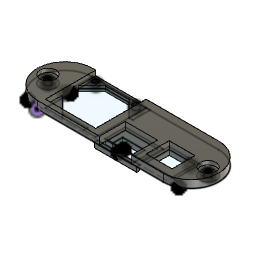
Complete_Housing_MyStat (Autodesk Fusion 360 archive; units mm, degrees)
design "MyStat Back Panel"
Autodesk Fusion 360 part; units mm, degrees
sketch "Sketch1" plane through (0, 0, 0) normal (0, 0, 1) x (1, 0, 0)
  line L0 (0, 0) -> (50, 0)
  line L1 (0, 22) -> (50, 22)
  arc A0 (0, 22) -> (0, 0) centre (0, 11) ccw
  arc A1 (50, 0) -> (50, 22) centre (50, 11) ccw
  circle A2 centre (-6.775, 11) radius 1.225
  circle A3 centre (56.775, 11) radius 1.225
  line L2 (-5, 1.202) -> (55, 1.202) construction
  line L3 (40.05, 12.3) -> (50.3, 12.3)
  line L4 (50.3, 12.3) -> (50.3, 3.2)
  line L5 (50.3, 3.2) -> (40.05, 3.2)
  line L6 (40.05, 3.2) -> (40.05, 12.3)
  line L7 (26.7, 7.2) -> (35.5, 7.2)
  line L8 (35.5, 7.2) -> (35.5, 3.2)
  line L9 (35.5, 3.2) -> (26.7, 3.2)
  line L10 (26.7, 3.2) -> (26.7, 7.2)
  line L11 (24.7, 3.2) -> (37.5, 3.2)
  line L12 (37.5, 3.2) -> (37.5, 10.2)
  line L13 (37.5, 10.2) -> (24.7, 10.2)
  line L14 (24.7, 10.2) -> (24.7, 3.2)
  line L15 (39.05, 3.2) -> (51.3, 3.2)
  line L16 (51.3, 3.2) -> (51.3, 13.3)
  line L17 (51.3, 13.3) -> (39.05, 13.3)
  line L18 (39.05, 13.3) -> (39.05, 3.2)
  line L19 (24.7, 1.202) -> (37.5, 1.202)
  line L20 (37.5, 1.202) -> (37.5, 0)
  line L21 (37.5, 0) -> (24.7, 0)
  line L22 (24.7, 0) -> (24.7, 1.202)
  line L23 (22.7, 1.202) -> (22.7, 0)
  line L24 (39.5, 1.202) -> (39.5, 0)
  line L25 (22.7, 1.202) -> (24.7, 1.202)
  line L26 (37.5, 1.202) -> (39.5, 1.202)
  line L27 (23.7, 3.2) -> (38.5, 3.2)
  line L28 (38.5, 3.2) -> (38.5, 11.2)
  line L29 (38.5, 11.2) -> (23.7, 11.2)
  line L30 (23.7, 11.2) -> (23.7, 3.2)
  line L31 (24.7, 3.2) -> (24.7, 1.202)
  line L32 (37.5, 3.2) -> (37.5, 1.202)
  line L33 (38.5, 3.2) -> (39.05, 3.2)
  line L34 (38.5, 11.2) -> (39.05, 11.2)
  circle A4 centre (-6.775, 11) radius 3.125
  circle A5 centre (56.775, 11) radius 3.125
  line L35 (1.2, 22) -> (21.2, 22)
  line L36 (21.2, 22) -> (21.2, 2)
  line L37 (21.2, 2) -> (1.2, 2)
  line L38 (1.2, 2) -> (1.2, 22)
  line L39 (7.9882, 22) -> (1.2, 15.2118)
  line L40 (14.4118, 22) -> (21.2, 15.2118)
  circle A6 centre (3.2, 20) radius 1.25
  circle A7 centre (19.2, 20) radius 1.25
  line L41 (6.4882, 20.5) -> (15.9118, 20.5)
  line L42 (21.2, 15.2118) -> (22.7, 15.2118)
  line L43 (22.7, 15.2118) -> (22.7, 22)
  line L44 (22.7, 22) -> (21.2, 22)
  line L45 (21.2, 22) -> (21.2, 15.2118)
  line L46 (1.2, 15.2118) -> (-0.3, 15.2118)
  line L47 (-0.3, 15.2118) -> (-0.3, 21.9959)
  line L48 (-0.3, 21.9959) -> (1.2, 21.9959)
  line L49 (1.2, 21.9959) -> (1.2, 15.2118)
  line L50 (1.2, 8.7882) -> (7.9882, 2)
  line L51 (6.4882, 3.5) -> (16.4882, 3.5)
  line L52 (16.4882, 3.5) -> (16.4882, 2)
  point P0 (-5, 1.202)
  point P1 (55, 1.202)
  point P2 (31.1, 1.202)
  point P3 (31.1, 3.2)
  point P4 (1.2, 12)
  dimension "d1" = 50
  dimension "d2" = 22
  dimension "d3" = 2.45
  dimension "d5" = 2.45
  dimension "d11" = 60
  dimension "d12" = 9.1
  dimension "d13" = 10.25
  dimension "d16" = 4.7
  dimension "d17" = 8.8
  dimension "d18" = 4
  dimension "d20" = 19.5
  dimension "d51" = 3
  dimension "d52" = 2
  dimension "d53" = 2
  dimension "d54" = 1
  dimension "d55" = 1
  dimension "d56" = 1
  dimension "d57" = 12.8
  dimension "d58" = 2
  dimension "d59" = 2
  dimension "d60" = 1
  dimension "d61" = 1
  dimension "d62" = 1
  dimension "d75" = 6.775
  dimension "d76" = 6.775
  dimension "d77" = 6.25
  dimension "d78" = 6.25
  dimension "d81" = 3.2
  dimension "d82" = 3.2
  dimension "d89" = 20
  dimension "d90" = 20
  dimension "d91" = 2.5
  dimension "d98" = 4.8
  dimension "d99" = 4.8
  dimension "d100" = 45
  dimension "d101" = 45
  dimension "d102" = 2.5
  dimension "d103" = 2.5
  dimension "d104" = 2
  dimension "d105" = 2
  dimension "d106" = 2
  dimension "d107" = 2
  dimension "d110" = 1.5
  dimension "d111" = 1.5
  dimension "d112" = 1.5
  dimension "d118" = 45
  dimension "d119" = 4.8
  dimension "d120" = 10
  dimension "d121" = 1.5
  constraint coincident L0.start A0.end
  constraint horizontal L0
  constraint horizontal L1
  constraint tangent L0 A0
  constraint tangent L1 A0
  constraint tangent L0 A1
  constraint tangent L1 A1
  constraint horizontal A0.centre A2.centre
  constraint horizontal A1.centre A3.centre
  constraint coincident A0 P0
  constraint coincident A1 P1
  constraint coincident P0 L2.start
  constraint coincident P1 L2.end
  constraint horizontal L2
  constraint horizontal L3
  constraint vertical L4
  constraint horizontal L5
  constraint vertical L6
  constraint horizontal L7
  constraint vertical L8
  constraint horizontal L9
  constraint vertical L10
  constraint horizontal L11
  constraint vertical L12
  constraint horizontal L13
  constraint vertical L14
  constraint collinear L9 L11
  constraint horizontal L15
  constraint vertical L16
  constraint horizontal L17
  constraint vertical L18
  constraint collinear L5 L15
  constraint horizontal L19
  constraint vertical L20
  constraint horizontal L21
  constraint vertical L22
  constraint coincident L0 L20.end
  constraint coincident L2 L19.start
  constraint midpoint L19 P2
  constraint midpoint L9 P3
  constraint vertical P2 P3
  constraint coincident L2 L23.start
  constraint coincident L0 L23.end
  constraint perpendicular L0 L23
  constraint coincident L2 L24.start
  constraint coincident L0 L24.end
  constraint perpendicular L0 L24
  constraint horizontal L27
  constraint vertical L28
  constraint horizontal L29
  constraint vertical L30
  constraint collinear L9 L27
  constraint coincident L18 L34.end
  constraint perpendicular L18 L34
  constraint concentric A2 A4
  constraint concentric A3 A5
  constraint horizontal L35
  constraint vertical L36
  constraint horizontal L37
  constraint vertical L38
  constraint coincident L35 L39.start
  constraint coincident L38 L39.end
  constraint coincident L35 L40.start
  constraint coincident L36 L40.end
  constraint collinear L1 L35
  constraint midpoint L38 P4
  constraint coincident L39 L41.start
  constraint coincident L40 L41.end
  constraint perpendicular L36 L41
  constraint horizontal L42
  constraint vertical L43
  constraint horizontal L44
  constraint vertical L45
  constraint coincident L1 L43.end
  constraint horizontal L46
  constraint vertical L47
  constraint horizontal L48
  constraint vertical L49
  constraint coincident A0 L47.end
  constraint coincident L38 L50.start
  constraint coincident L37 L50.end
  constraint coincident L50 L51.start
  constraint perpendicular L36 L51
  constraint coincident L37 L52.end
  constraint perpendicular L37 L52
  measures "d1" distance of L0.start L0.end
  measures "d2" distance of L0 L1
  measures "d3" diameter of A2
  measures "d5" diameter of A3
  measures "d11" distance of P0 P1
  measures "d12" distance of L3 L5
  measures "d13" distance of L4 L6
  measures "d16" distance of P1 L4
  measures "d17" distance of L7.start L7.end
  measures "d18" distance of L7.start L9.end
  measures "d20" distance of P1 L8
  measures "d51" distance of L7 L13
  measures "d52" distance of L10 L14
  measures "d53" distance of L8 L12
  measures "d54" distance of L6 L18
  measures "d55" distance of L3 L17
  measures "d56" distance of L4 L16
  measures "d57" distance of L20 L22
  measures "d58" distance of L22 L23
  measures "d59" distance of L20 L24
  measures "d60" distance of L14 L30
  measures "d61" distance of L13 L29
  measures "d62" distance of L12 L28
  measures "d75" distance of A0.centre A2.centre
  measures "d76" distance of A1.centre A3.centre
  measures "d77" diameter of A4
  measures "d78" diameter of A5
  measures "d81" distance of L0 L9
  measures "d82" distance of L0 L5
  measures "d89" distance of L35.start L35.end
  measures "d90" distance of L35.start L37.end
  measures "d91" distance of L30 L36
  measures "d98" distance of L35.start L39
  measures "d99" distance of L35.end L40
  measures "d100" angle of L38 L39
  measures "d101" angle of L36 L40
  measures "d102" diameter of A6
  measures "d103" diameter of A7
  measures "d104" distance of L38 A6.centre
  measures "d105" distance of L35 A6.centre
  measures "d106" distance of L35 A7.centre
  measures "d107" distance of L36 A7.centre
  measures "d110" distance of L1 L41
  measures "d111" distance of L40.end L42.end
  measures "d112" distance of L39.end L46.end
  measures "d118" angle of L37 L50
  measures "d119" distance of L37.end L50
  measures "d120" distance of L51.start L51.end
  measures "d121" distance of L51.end L52.end
extrude "Extrude16" add sketch "Sketch1" along normal blind 3 contours L0 L1 A0 A1 L5 L15 L16 L17 L18 L23 L24 L25 L26 L27 L29 L30 L31 L32 L33 L34 L36 L37 L38 L42 L43 L46 L47 | L0 L22 L23 L25 | L38 L46 L47 L48 L49 | L1 A0 L38 L48 | L1 L35 L38 L39 L49 | L0 L20 L24 L26 | L36 L37 L38 L39 L40 L41 L50 L51 L52 | L12 L13 L14 L27 L28 L29 L30 | L1 L35 L39 L40 L41 | L37 L38 L50 | L1 L35 L36 L40 L45 | L37 L50 L51 L52 | L18 L28 L33 L34 | L1 L36 L42 L43 L44 L45 | L3 L4 L6 L15 L16 L17 L18 | A6 | A7
extrude "Extrude17" add sketch "Sketch1" against normal blind 2 contours L0 L22 L23 L25 | L0 L19 L20 L21 L22 | L0 L20 L24 L26 | L7 L8 L10 L11 L12 L13 L14 L27 | L12 L13 L14 L27 L28 L29 L30 | L3 L4 L6 L15 L16 L17 L18
extrude "Extrude18" add sketch "Sketch1" along normal blind 1.5 contours A4 | A5
extrude "Extrude19" cut sketch "Sketch1" along normal blind 3 contours L1 L35 L38 L39 L49 | L36 L37 L38 L39 L40 L41 L50 L51 L52 | L1 L35 L39 L40 L41 | L37 L38 L50 | L1 L35 L36 L40 L45 | L37 L50 L51 L52 | A6 | A7
extrude "Extrude20" add sketch "Sketch1" along normal blind 1 and the other way blind 1 contours L1 L35 L38 L39 L49 | L1 L35 L39 L40 L41 | L1 L35 L36 L40 L45
extrude "Extrude21" add sketch "Sketch1" against normal blind 1 contours L38 L46 L47 L48 L49 | L1 L36 L42 L43 L44 L45
extrude "Extrude23" add sketch "Sketch1" along normal blind 1 contours L37 L38 L50 | L37 L50 L51 L52
equation "d76 = d75"
equation "d82 = d81"

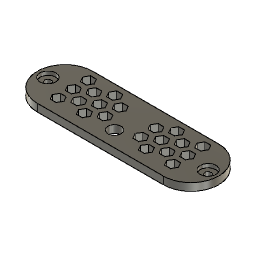
design "MyStat Front Panel 2.5"
Autodesk Fusion 360 part; units mm, degrees
sketch "Sketch1" plane through (0, 0, 0) normal (0, 0, 1) x (1, 0, 0)
  line L0 (0, 0) -> (50, 0)
  line L1 (0, 22) -> (50, 22)
  arc A0 (0, 22) -> (0, 0) centre (0, 11) ccw
  arc A1 (50, 0) -> (50, 22) centre (50, 11) ccw
  circle A2 centre (-6.775, 11) radius 1.225
  circle A3 centre (56.775, 11) radius 1.225
  circle A4 centre (24.5, 6.15) radius 2.6
  line L2 (-5, 1.202) -> (55, 1.202) construction
  circle A5 centre (-6.775, 11) radius 3.125
  circle A6 centre (56.775, 11) radius 3.125
  line L3 (4.6188, 18) -> (3.4641, 20)
  line L4 (3.4641, 20) -> (1.1547, 20)
  line L5 (1.1547, 20) -> (0, 18)
  line L6 (0, 18) -> (1.1547, 16)
  line L7 (1.1547, 16) -> (3.4641, 16)
  line L8 (3.4641, 16) -> (4.6188, 18)
  line L9 (0, 22) -> (0, 0) construction
  line L10 (50, 22) -> (50, 0) construction
  line L11 (4.6188, 12) -> (3.4641, 14)
  line L12 (3.4641, 14) -> (1.1547, 14)
  line L13 (1.1547, 10) -> (3.4641, 10)
  line L14 (3.4641, 10) -> (4.6188, 12)
  line L15 (1.1547, 14) -> (0, 12)
  line L16 (0, 12) -> (1.1547, 10)
  line L17 (4.6188, 6) -> (3.4641, 8)
  line L18 (3.4641, 8) -> (1.1547, 8)
  line L19 (1.1547, 4) -> (3.4641, 4)
  line L20 (3.4641, 4) -> (4.6188, 6)
  line L21 (1.1547, 8) -> (0, 6)
  line L22 (0, 6) -> (1.1547, 4)
  line L23 (9.815, 15) -> (8.6603, 17)
  line L24 (8.6603, 17) -> (6.3509, 17)
  line L25 (6.3509, 13) -> (8.6603, 13)
  line L26 (8.6603, 13) -> (9.815, 15)
  line L27 (6.3509, 17) -> (5.1962, 15)
  line L28 (5.1962, 15) -> (6.3509, 13)
  line L29 (9.815, 9) -> (8.6603, 11)
  line L30 (8.6603, 11) -> (6.3509, 11)
  line L31 (6.3509, 7) -> (8.6603, 7)
  line L32 (8.6603, 7) -> (9.815, 9)
  line L33 (6.3509, 11) -> (5.1962, 9)
  line L34 (5.1962, 9) -> (6.3509, 7)
  line L35 (15.0111, 12) -> (13.8564, 14)
  line L36 (13.8564, 14) -> (11.547, 14)
  line L37 (11.547, 10) -> (13.8564, 10)
  line L38 (13.8564, 10) -> (15.0111, 12)
  line L39 (11.547, 14) -> (10.3923, 12)
  line L40 (10.3923, 12) -> (11.547, 10)
  line L41 (15.0111, 6) -> (13.8564, 8)
  line L42 (11.547, 4) -> (13.8564, 4)
  line L43 (11.547, 8) -> (10.3923, 6)
  line L44 (13.8564, 8) -> (11.547, 8)
  line L45 (10.3923, 6) -> (11.547, 4)
  line L46 (13.8564, 4) -> (15.0111, 6)
  line L47 (20.2073, 15) -> (19.0526, 17)
  line L48 (16.7432, 13) -> (19.0526, 13)
  line L49 (16.7432, 17) -> (15.5885, 15)
  line L50 (19.0526, 17) -> (16.7432, 17)
  line L51 (15.5885, 15) -> (16.7432, 13)
  line L52 (19.0526, 13) -> (20.2073, 15)
  line L53 (15.0111, 18) -> (13.8564, 20)
  line L54 (11.547, 16) -> (13.8564, 16)
  line L55 (11.547, 20) -> (10.3923, 18)
  line L56 (13.8564, 20) -> (11.547, 20)
  line L57 (10.3923, 18) -> (11.547, 16)
  line L58 (13.8564, 16) -> (15.0111, 18)
  line L59 (15.5885, 9) -> (16.7432, 7)
  line L60 (19.0526, 7) -> (20.2073, 9)
  line L61 (16.7432, 11) -> (15.5885, 9)
  line L62 (19.0526, 11) -> (16.7432, 11)
  line L63 (20.2073, 9) -> (19.0526, 11)
  line L64 (16.7432, 7) -> (19.0526, 7)
  line L65 (25, 22) -> (25, 0) construction
  line L66 (50, 6) -> (48.8453, 4)
  line L67 (48.8453, 4) -> (46.5359, 4)
  line L68 (46.5359, 14) -> (48.8453, 14)
  line L69 (41.3397, 11) -> (43.6491, 11)
  line L70 (38.453, 10) -> (36.1436, 10)
  line L71 (48.8453, 16) -> (46.5359, 16)
  line L72 (48.8453, 10) -> (46.5359, 10)
  line L73 (40.185, 9) -> (41.3397, 11)
  line L74 (36.1436, 8) -> (38.453, 8)
  line L75 (33.2568, 7) -> (30.9474, 7)
  line L76 (48.8453, 20) -> (50, 18)
  line L77 (50, 12) -> (48.8453, 10)
  line L78 (33.2568, 13) -> (30.9474, 13)
  line L79 (30.9474, 13) -> (29.7927, 15)
  line L80 (30.9474, 7) -> (29.7927, 9)
  line L81 (30.9474, 11) -> (33.2568, 11)
  line L82 (41.3397, 7) -> (40.185, 9)
  line L83 (46.5359, 8) -> (48.8453, 8)
  line L84 (29.7927, 15) -> (30.9474, 17)
  line L85 (29.7927, 9) -> (30.9474, 11)
  line L86 (34.9889, 6) -> (36.1436, 8)
  line L87 (46.5359, 20) -> (48.8453, 20)
  line L88 (43.6491, 7) -> (41.3397, 7)
  line L89 (33.2568, 11) -> (34.4115, 9)
  line L90 (48.8453, 8) -> (50, 6)
  line L91 (46.5359, 10) -> (45.3812, 12)
  line L92 (50, 18) -> (48.8453, 16)
  line L93 (34.4115, 9) -> (33.2568, 7)
  line L94 (36.1436, 10) -> (34.9889, 12)
  line L95 (39.6077, 12) -> (38.453, 10)
  line L96 (38.453, 8) -> (39.6077, 6)
  line L97 (39.6077, 6) -> (38.453, 4)
  line L98 (45.3812, 6) -> (46.5359, 8)
  line L99 (34.9889, 12) -> (36.1436, 14)
  line L100 (38.453, 14) -> (39.6077, 12)
  line L101 (38.453, 20) -> (39.6077, 18)
  line L102 (36.1436, 20) -> (38.453, 20)
  line L103 (36.1436, 4) -> (34.9889, 6)
  line L104 (38.453, 4) -> (36.1436, 4)
  line L105 (46.5359, 4) -> (45.3812, 6)
  line L106 (40.185, 15) -> (41.3397, 17)
  line L107 (44.8038, 9) -> (43.6491, 7)
  line L108 (36.1436, 16) -> (34.9889, 18)
  line L109 (38.453, 16) -> (36.1436, 16)
  line L110 (43.6491, 17) -> (44.8038, 15)
  line L111 (39.6077, 18) -> (38.453, 16)
  line L112 (44.8038, 15) -> (43.6491, 13)
  line L113 (41.3397, 17) -> (43.6491, 17)
  line L114 (45.3812, 18) -> (46.5359, 20)
  line L115 (34.9889, 18) -> (36.1436, 20)
  line L116 (41.3397, 13) -> (40.185, 15)
  line L117 (43.6491, 13) -> (41.3397, 13)
  line L118 (36.1436, 14) -> (38.453, 14)
  line L119 (34.4115, 15) -> (33.2568, 13)
  line L120 (33.2568, 17) -> (34.4115, 15)
  line L121 (46.5359, 16) -> (45.3812, 18)
  line L122 (45.3812, 12) -> (46.5359, 14)
  line L123 (43.6491, 11) -> (44.8038, 9)
  line L124 (30.9474, 17) -> (33.2568, 17)
  line L125 (48.8453, 14) -> (50, 12)
  point P0 (-5, 1.202)
  point P1 (55, 1.202)
  point P2 (2.3094, 18)
  point P3 (2.3094, 12)
  point P4 (2.3094, 6)
  point P5 (7.5056, 15)
  point P6 (7.5056, 9)
  point P7 (12.7017, 12)
  point P8 (12.7017, 6)
  point P9 (17.8979, 15)
  point P10 (12.7017, 18)
  point P11 (17.8979, 9)
  point P12 (42.4944, 9)
  point P13 (37.2983, 6)
  point P14 (32.1021, 9)
  point P15 (47.6906, 6)
  point P16 (37.2983, 12)
  point P17 (32.1021, 15)
  point P18 (37.2983, 18)
  point P19 (47.6906, 12)
  point P20 (47.6906, 18)
  point P21 (42.4944, 15)
  point P22 (50, 11)
  dimension "d1" = 50
  dimension "d2" = 22
  dimension "d3" = 50
  dimension "d5" = 2.45
  dimension "d6" = 2.45
  dimension "d10" = 60
  dimension "d11" = 30.5
  dimension "d12" = 5.2
  dimension "d24" = 6.775
  dimension "d25" = 6.775
  dimension "d26" = 6.25
  dimension "d27" = 6.25
  dimension "d32" = 6.15
  dimension "d33" = 2
  dimension "d34" = 2
  dimension "d35" = 2
  dimension "d36" = 2
  dimension "d37" = 2
  dimension "d38" = 2
  dimension "d39" = 2
  dimension "d40" = 2
  dimension "d41" = 2
  dimension "d42" = 2
  dimension "d43" = 2
  dimension "d44" = 2
  dimension "d45" = 2
  dimension "d47" = 2
  dimension "d48" = 2
  dimension "d49" = 2
  dimension "d50" = 2
  dimension "d51" = 2
  dimension "d52" = 2
  dimension "d53" = 2
  dimension "d54" = 2
  dimension "d55" = 2
  dimension "d56" = 2
  dimension "d58" = 2
  dimension "d59" = 2
  dimension "d60" = 2
  dimension "d61" = 2
  constraint coincident L0.start A0.end
  constraint horizontal L0
  constraint horizontal L1
  constraint tangent L1 A0
  constraint tangent L0 A1
  constraint tangent L1 A1
  constraint horizontal A0.centre A2.centre
  constraint horizontal P22 A3.centre
  constraint coincident A0 P0
  constraint coincident A1 P1
  constraint horizontal P0 P1
  constraint coincident P0 L2.start
  constraint coincident P1 L2.end
  constraint concentric A2 A5
  constraint concentric A3 A6
  constraint coincident L5.end L9
  constraint coincident L9 L15.end
  constraint coincident L9 L21.end
  constraint midpoint L1 L65.start
  constraint midpoint L0 L65.end
  constraint symmetric A0.centre L65 P22
  constraint symmetric L3.start L65 L114.start
  constraint symmetric L3.end L65 L87.start
  constraint symmetric L4.end L65 L76.start
  constraint symmetric L5.end L65 L76.end
  constraint symmetric L6.end L65 L71.start
  constraint symmetric L7.end L65 L71.end
  constraint symmetric P2 L65 P20
  constraint symmetric L11.start L65 L91.end
  constraint symmetric L15.end L65 L77.start
  constraint symmetric L12.end L65 L68.end
  constraint symmetric L13.start L65 L72.start
  constraint symmetric L11.end L65 L68.start
  constraint symmetric L13.end L65 L72.end
  constraint symmetric P3 L65 P19
  constraint symmetric L17.start L65 L98.start
  constraint symmetric L21.end L65 L66.start
  constraint symmetric L18.end L65 L83.end
  constraint symmetric L19.start L65 L66.end
  constraint symmetric L17.end L65 L83.start
  constraint symmetric L19.end L65 L67.end
  constraint symmetric P4 L65 P15
  constraint symmetric L23.start L65 L106.start
  constraint symmetric L27.end L65 L110.end
  constraint symmetric L24.end L65 L110.start
  constraint symmetric L25.start L65 L112.end
  constraint symmetric L23.end L65 L106.end
  constraint symmetric L25.end L65 L116.start
  constraint symmetric P5 L65 P21
  constraint symmetric L29.start L65 L73.start
  constraint symmetric L33.end L65 L107.start
  constraint symmetric L30.end L65 L69.end
  constraint symmetric L31.start L65 L88.start
  constraint symmetric L29.end L65 L69.start
  constraint symmetric L31.end L65 L82.start
  constraint symmetric P6 L65 P12
  constraint symmetric L35.start L65 L94.end
  constraint symmetric L39.end L65 L95.start
  constraint symmetric L36.end L65 L100.start
  constraint symmetric L37.start L65 L70.start
  constraint symmetric L35.end L65 L99.end
  constraint symmetric L37.end L65 L70.end
  constraint symmetric P7 L65 P16
  constraint symmetric L41.start L65 L86.start
  constraint symmetric L43.end L65 L96.end
  constraint symmetric L43.start L65 L74.end
  constraint symmetric L42.start L65 L97.end
  constraint symmetric L41.end L65 L74.start
  constraint symmetric L42.end L65 L103.start
  constraint symmetric P8 L65 P13
  constraint symmetric L47.start L65 L79.end
  constraint symmetric L49.end L65 L119.start
  constraint symmetric L49.start L65 L120.start
  constraint symmetric L48.start L65 L78.start
  constraint symmetric L47.end L65 L84.end
  constraint symmetric L48.end L65 L78.end
  constraint symmetric P9 L65 P17
  constraint symmetric L53.start L65 L108.end
  constraint symmetric L55.end L65 L101.end
  constraint symmetric L55.start L65 L101.start
  constraint symmetric L54.start L65 L109.start
  constraint symmetric L53.end L65 L102.start
  constraint symmetric L54.end L65 L108.start
  constraint symmetric P10 L65 P18
  constraint symmetric L59.start L65 L89.end
  constraint symmetric L61.start L65 L81.end
  constraint symmetric L59.end L65 L75.start
  constraint symmetric L62.start L65 L81.start
  constraint symmetric L60.start L65 L75.end
  constraint symmetric P11 L65 P14
  constraint symmetric L60.end L65 L80.end
  measures "d1" distance of L0.start L0.end
  measures "d2" distance of L0 L1
  measures "d3" distance of L1.start L1.end
  measures "d5" diameter of A2
  measures "d6" diameter of A3
  measures "d10" horizontal distance of P0 P1
  measures "d11" horizontal distance of P1 A4.centre
  measures "d12" diameter of A4
  measures "d24" distance of A0.centre A2.centre
  measures "d25" distance of P22 A3.centre
  measures "d26" diameter of A5
  measures "d27" diameter of A6
  measures "d32" distance of L0 A4.centre
  measures "d33" distance of P2 L8
  measures "d34" distance of L1 L4
  measures "d35" distance of P3 L14
  measures "d36" distance of P4 L20
  measures "d37" distance of P5 L26
  measures "d38" distance of P6 L32
  measures "d39" distance of P7 L38
  measures "d40" distance of L7 L12
  measures "d41" distance of L13 L18
  measures "d42" distance of L8 L27
  measures "d43" distance of L11 L28
  measures "d44" distance of L14 L33
  measures "d45" distance of L17 L34
  measures "d47" distance of P8 L46
  measures "d48" distance of P9 L52
  measures "d49" distance of P10 L58
  measures "d50" distance of L26 L39
  measures "d51" distance of L29 L40
  measures "d52" distance of L23 L57
  measures "d53" distance of L36 L54
  measures "d54" distance of L32 L43
  measures "d55" distance of L37 L44
  measures "d56" distance of P11 L60
  measures "d58" distance of L41 L59
  measures "d59" distance of L38 L61
  measures "d60" distance of L35 L51
  measures "d61" distance of L49 L58
extrude "Extrude3" add sketch "Sketch1" along normal blind 3 contours L0 L1 A0 A1 | L3 L4 L5 L6 L7 L8 | L11 L12 L13 L14 L15 L16 | L17 L18 L19 L20 L21 L22 | L23 L24 L25 L26 L27 L28 | L29 L30 L31 L32 L33 L34 | L35 L36 L37 L38 L39 L40 | L41 L42 L43 L44 L45 L46 | L47 L48 L49 L50 L51 L52 | L53 L54 L55 L56 L57 L58 | L59 L60 L61 L62 L63 L64 | L66 L67 L83 L90 L98 L105 | L68 L72 L77 L91 L122 L125 | L69 L73 L82 L88 L107 L123 | L70 L94 L95 L99 L100 L118 | L71 L76 L87 L92 L114 L121 | L74 L86 L96 L97 L103 L104 | L75 L80 L81 L85 L89 L93 | L78 L79 L84 L119 L120 L124 | L101 L102 L108 L109 L111 L115 | L106 L110 L112 L113 L116 L117
extrude "Extrude4" add sketch "Sketch1" along normal blind 1.5 contours A5 | A6
extrude "Extrude5" cut sketch "Sketch1" along normal blind 3 contours L3 L4 L5 L6 L7 L8 | L11 L12 L13 L14 L15 L16 | L17 L18 L19 L20 L21 L22 | L23 L24 L25 L26 L27 L28 | L29 L30 L31 L32 L33 L34 | L35 L36 L37 L38 L39 L40 | L41 L42 L43 L44 L45 L46 | L47 L48 L49 L50 L51 L52 | L53 L54 L55 L56 L57 L58 | L59 L60 L61 L62 L63 L64 | L66 L67 L83 L90 L98 L105 | L68 L72 L77 L91 L122 L125 | L69 L73 L82 L88 L107 L123 | L70 L94 L95 L99 L100 L118 | L71 L76 L87 L92 L114 L121 | L74 L86 L96 L97 L103 L104 | L75 L80 L81 L85 L89 L93 | L78 L79 L84 L119 L120 L124 | L101 L102 L108 L109 L111 L115 | L106 L110 L112 L113 L116 L117
equation "d3 = d1"
equation "d25 = d24"
equation "d27 = d26"
